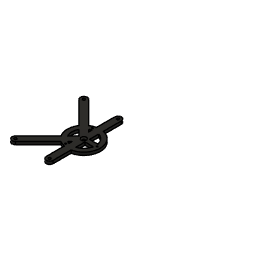
sensors-plate_lidar2d_ldrobot-d300-ld19_support (Autodesk Fusion 360 design; units mm, degrees)
Autodesk Fusion 360 part; units mm, degrees
sketch "Sketch1" plane through (0, 392, 0) normal (0, 1, 0) x (-1, 0, 0)
  circle A0 centre (120, -60) radius 2
  circle A1 centre (0, 120) radius 2
  circle A2 centre (120, 120) radius 2
  circle A3 centre (-120, 0) radius 2
  circle A4 centre (0, -120) radius 2
  circle A5 centre (0, -60) radius 2
  circle A6 centre (165.5, 26.5835) radius 2.5
  circle A7 centre (0, 0) radius 2
  circle A8 centre (60, 120) radius 2
  circle A9 centre (-165.5, -26.5835) radius 2.5
  circle A10 centre (165.5, 78.1855) radius 2.5
  circle A11 centre (120, 0) radius 2
  circle A12 centre (120, -120) radius 2
  circle A13 centre (-60, 60) radius 2
  circle A14 centre (-60, 120) radius 2
  circle A15 centre (-120, -60) radius 2
  circle A16 centre (60, 60) radius 2
  circle A17 centre (0, 60) radius 2
  circle A18 centre (165.5, -26.5835) radius 2.5
  circle A19 centre (60, -60) radius 2
  circle A20 centre (-165.5, 26.5835) radius 2.5
  circle A21 centre (60, 0) radius 2
  circle A22 centre (120, 60) radius 2
  circle A23 centre (165.5, -78.1855) radius 2.5
  circle A24 centre (-120, 60) radius 2
  circle A25 centre (-120, 120) radius 2
  circle A26 centre (-60, -120) radius 2
  circle A27 centre (-165.5, 78.1855) radius 2.5
  circle A28 centre (-120, -120) radius 2
  circle A29 centre (-60, 0) radius 2
  circle A30 centre (60, -120) radius 2
  circle A31 centre (-165.5, -78.1855) radius 2.5
  circle A32 centre (-60, -60) radius 2
  line L0 (-176, 131) -> (-176, -131)
  line L1 (-176, -131) -> (176, -131)
  line L2 (176, -131) -> (176, 131)
  line L3 (176, 131) -> (-176, 131)
  circle A33 centre (-120, 60) radius 6
  circle A34 centre (-120, 0) radius 6
  circle A35 centre (-120, -60) radius 6
  circle A36 centre (-60, -60) radius 6
  circle A37 centre (-60, 60) radius 6
  circle A38 centre (-120, 60) radius 2.15
  circle A39 centre (-120, 0) radius 2.15
  circle A40 centre (-120, -60) radius 2.15
  circle A41 centre (-60, -60) radius 2.15
  circle A42 centre (-60, 60) radius 2.15
  line L4 (-126, -60) -> (-126, 60)
  line L5 (-64.2426, 64.2426) -> (-124.2426, 4.2426)
  line L6 (-115.7574, -4.2426) -> (-55.7574, 55.7574)
  line L7 (-55.7574, -55.7574) -> (-115.7574, 4.2426)
  line L8 (-64.2426, -64.2426) -> (-124.2426, -4.2426)
  line L9 (-114, 60) -> (-114, -60)
  circle A43 centre (-120, 0) radius 17.5 construction
  line L10 (-139.295, 19.295) -> (-100.705, 19.295) construction
  line L11 (-100.705, 19.295) -> (-100.705, -19.295) construction
  line L12 (-100.705, -19.295) -> (-139.295, -19.295) construction
  line L13 (-139.295, -19.295) -> (-139.295, 19.295) construction
  line L14 (-139.295, 19.295) -> (-100.705, -19.295) construction
  line L15 (-100.705, 19.295) -> (-139.295, -19.295) construction
  line L16 (-100.705, 0) -> (-176, 0) construction
  circle A44 centre (-143.42, 0) radius 1.25
  line L17 (-120, 0) -> (-120, 19.295) construction
  line L18 (-120, 0) -> (-120, -19.295) construction
  circle A45 centre (-111.5, 23.4) radius 1.4
  circle A46 centre (-111.5, -23.4) radius 1.4
  circle A47 centre (-120, 0) radius 24.896 construction
  circle A48 centre (-120, 0) radius 28.896
  circle A49 centre (-120, 0) radius 20.896
  circle A50 centre (-143.42, 0) radius 4 construction
  circle A51 centre (-120, 0) radius 4 construction
  line L19 (-143.42, 4) -> (-120, 4)
  line L20 (-120, -4) -> (-143.42, -4)
  point P0 (-120, 0)
  dimension "d271" = 12
  dimension "d272" = 0.15
  dimension "d273" = 0.15
  dimension "d274" = 0.15
  dimension "d275" = 0.15
  dimension "d276" = 0.15
  dimension "d277" = 35
  dimension "d278" = 38.59
  dimension "d280" = 2.5
  dimension "d281" = 42.715
  dimension "d282" = 27.795
  dimension "d283" = 2.8
  dimension "d284" = 46.8
  dimension "d285" = 4
  dimension "d286" = -4
  dimension "d287" = 8
  dimension "d288" = 8
  constraint concentric A24 A33
  constraint concentric A3 A34
  constraint concentric A15 A35
  constraint concentric A32 A36
  constraint concentric A13 A37
  constraint equal A33 A34
  constraint equal A33 A37
  constraint equal A33 A35
  constraint equal A33 A36
  constraint coincident A35 L4.start
  constraint coincident A33 L4.end
  constraint coincident A37 L5.start
  constraint coincident A34 L5.end
  constraint coincident A34 L6.start
  constraint coincident A37 L6.end
  constraint coincident A36 L7.start
  constraint coincident A34 L7.end
  constraint tangent A34 L7
  constraint coincident A36 L8.start
  constraint coincident A34 L8.end
  constraint tangent A33 L4
  constraint tangent A35 L4
  constraint tangent A37 L5
  constraint tangent A37 L6
  constraint tangent A34 L5
  constraint tangent A34 L6
  constraint tangent A34 L8
  constraint tangent A36 L7
  constraint tangent A36 L8
  constraint coincident A33 L9.start
  constraint coincident A35 L9.end
  constraint tangent A33 L9
  constraint tangent A35 L9
  constraint concentric A34 A43
  constraint horizontal L10
  constraint perpendicular L10 L11
  constraint parallel L10 L12
  constraint parallel L11 L13
  constraint coincident L14 P0
  constraint coincident L15 P0
  constraint coincident P0 A3.centre
  constraint equal L10 L11
  constraint midpoint L11 L16.start
  constraint midpoint L0 L16.end
  constraint coincident L16 A44.centre
  constraint midpoint L10 L17.end
  constraint midpoint L12 L18.end
  constraint symmetric L16 A45 A46
  constraint concentric A34 A47
  constraint coincident A45.centre A47
  constraint concentric A44 A50
  constraint concentric A34 A51
  constraint coincident A50 L19.start
  constraint coincident A51 L19.end
  constraint coincident A51 L20.start
  constraint coincident A50 L20.end
  constraint tangent A51 L19
  constraint tangent A51 L20
  constraint tangent A50 L20
  constraint tangent A50 L19
  measures "d271" diameter of A33
  measures "d277" diameter of A43
  measures "d278" distance of L11.end L12.end
  measures "d280" diameter of A44
  measures "d281" distance of L11 A44.centre
  measures "d282" distance of L13 A45.centre
  measures "d283" diameter of A45
  measures "d284" distance of A45.centre A46.centre
  measures "d287" diameter of A50
  measures "d288" diameter of A51
extrude "Extrude1" add sketch "Sketch1" along normal blind 5 contours A33 | A33 L4 L9 A48 | L5 L9 A48 A49 | L4 L9 A48 A49 | L4 A48 A49 | A34 L4 L5 L9 A49 L19 | L5 L6 A48 A49 | A37 L5 L6 A48 | A35 L4 L9 A48 | L4 L9 A48 A49 | A34 L5 L7 L9 | L5 L6 L7 L9 A49 | A37 | L6 L7 A48 A49 | A34 L4 L19 | L4 A49 L19 L20 | A35 | A34 L4 L8 L9 A49 L20 | L8 L9 A48 A49 | A34 | A34 L7 L9 | L6 L7 L9 | A34 L4 L20 | A36 L7 L8 A48 | L7 L8 A48 A49 | L6 L7 L8 L9 A49 | A34 L6 L9 | A34 L6 L8 L9 | A36
hole "Hole1" at (120, 397, 0) direction (0, -1, 0) diameter 4 depth 5 tip angle 180 countersink diameter 9 countersink angle 90
hole "Hole2" at (111.5, 392, 23.4) direction (0, 1, 0) diameter 2.5 depth 5 tip angle 180 countersink diameter 6 countersink angle 90
hole "Hole3" at (111.5, 392, -23.4) direction (0, 1, 0) diameter 2.5 depth 5 tip angle 180 countersink diameter 6 countersink angle 90
hole "Hole4" at (143.42, 392, 0) direction (0, 1, 0) diameter 2.5 depth 5 tip angle 180 countersink diameter 6 countersink angle 90
